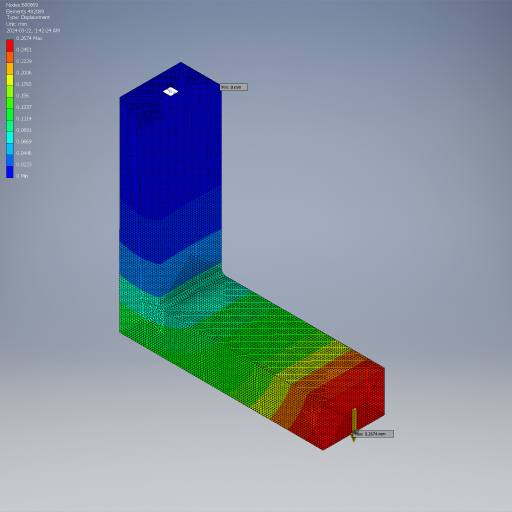
# Autodesk Inventor part: CE-10.1.3
Saved by Autodesk Inventor 2024 (Build 280153000, 153)
## iProperties
Created: 2024-03-22
Part Number: CE-10.1.3
Material: Stainless Steel
Document SubType Name: Modeling
Designer: Alex
Density: 8 g/cm^3
Appearance: Semi-Polished
Author: Alex
Autodesk Inventor part; units mm, degrees
ref_plane "YZ Plane" through (0, 0, 0) normal (1, 0, 0) x (0, 1, 0)
ref_plane "XZ Plane" through (0, 0, 0) normal (0, 1, 0) x (-1, 0, 0)
ref_plane "XY Plane" through (0, 0, 0) normal (0, 0, 1) x (1, 0, 0)
sketch "Sketch1" plane through (0, 0, 0) normal (0, 0, 1) x (1, 0, 0)
  line L0 (0, 0) -> (100, 0)
  line L1 (100, 0) -> (100, 20)
  line L2 (0, 0) -> (0, 100)
  line L3 (0, 100) -> (20, 100)
  line L4 (20, 100) -> (20, 20)
  line L5 (20, 20) -> (100, 20)
  dimension "d0" = 100
  dimension "d1" = 20
  dimension "d2" = 100
  dimension "d3" = 20
  constraints: 12 end point, 4 perpendicular, 1 horizontal, 1 vertical
  measures "d0" distance of L0.start L0.end
  measures "d1" distance of L0.end L1.end
  measures "d2" distance of L0.start L2.end
  measures "d3" distance of L2.end L3.end
extrude "Extrusion1" add sketch "Sketch1" along normal mid plane 30
fillet "Fillet1" radius 2 1 edges at (20, 20, 0)
body "Solid1"
